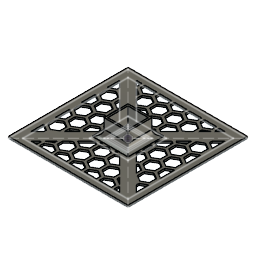
base (Autodesk Fusion 360 design; units mm, degrees)
Autodesk Fusion 360 part; units mm, degrees
(part 1 of 2)
sketch "Sketch4" plane through (0, 0, 0) normal (0, 0, 1) x (1, 0, 0)
  line L0 (100, -100) -> (-100, -100)
  line L1 (-100, -100) -> (-100, 100)
  line L2 (-100, 100) -> (100, 100)
  line L3 (100, 100) -> (100, -100)
  line L4 (100, -100) -> (-100, 100) construction
  line L5 (-100, -100) -> (100, 100) construction
  line L6 (20, -20) -> (-20, -20)
  line L7 (-20, -20) -> (-20, 20)
  line L8 (-20, 20) -> (20, 20)
  line L9 (20, 20) -> (20, -20)
  line L10 (20, -20) -> (-20, 20) construction
  line L11 (-20, -20) -> (20, 20) construction
  line L12 (-32, -32) -> (-32, 32)
  line L13 (-32, 32) -> (32, 32)
  line L14 (32, 32) -> (32, -32)
  line L15 (32, -32) -> (-32, -32)
  line L16 (88, -88) -> (-88, -88)
  line L17 (-88, -88) -> (-88, 88)
  line L18 (-88, 88) -> (88, 88)
  line L19 (88, 88) -> (88, -88)
  line L20 (17, 17) -> (17, -17)
  line L21 (17, -17) -> (-17, -17)
  line L22 (-17, -17) -> (-17, 17)
  line L23 (-17, 17) -> (17, 17)
  line L24 (14, -14) -> (-14, -14)
  line L25 (-14, -14) -> (-14, 14)
  line L26 (-14, 14) -> (14, 14)
  line L27 (14, 14) -> (14, -14)
  line L28 (-73.8579, 88) -> (-17.8579, 32)
  line L29 (-88, 73.8579) -> (-32, 17.8579)
  dimension "d22" = 200
  dimension "d23" = 200
  dimension "d24" = 40
  dimension "d25" = 40
  dimension "d26" = -12
  dimension "d27" = 12
  dimension "d44" = 3
  dimension "d49" = 6
  dimension "d50" = 20
  constraint horizontal L0
  constraint perpendicular L0 L1
  constraint parallel L0 L2
  constraint parallel L1 L3
  constraint coincident L4 origin
  constraint coincident L5 origin
  constraint horizontal L6
  constraint perpendicular L6 L7
  constraint parallel L6 L8
  constraint parallel L7 L9
  constraint coincident L10 origin
  constraint coincident L11 origin
  constraint coincident L18 L28.start
  constraint coincident L13 L28.end
  constraint coincident L17 L29.start
  constraint coincident L12 L29.end
  constraint parallel L4 L29
  constraint symmetric L4 L28 L29
  measures "d22" distance of L1.end L2.end
  measures "d23" distance of L0.end L1.end
  measures "d24" distance of L7.end L8.end
  measures "d25" distance of L6.end L7.end
  measures "d50" distance of L28 L29
extrude "Extrude4" add sketch "Sketch4" along normal blind 3 contours L0 L1 L2 L3 | L6 L7 L8 L9 | L12 L13 L14 L15 | L20 L21 L22 L23 | L24 L25 L26 L27 makes body 1 at (-96, -29.3333, 0) makes body 2 at (10.6667, -10.6667, 0)
sketch "Sketch6" plane through (0, 0, 0) normal (0, 0, 1) x (1, 0, 0)
  line L0 (10, 5.7735) -> (0, 11.547)
  line L1 (0, 11.547) -> (-10, 5.7735)
  line L2 (-10, 5.7735) -> (-10, -5.7735)
  line L3 (-10, -5.7735) -> (0, -11.547)
  line L4 (0, -11.547) -> (10, -5.7735)
  line L5 (10, -5.7735) -> (10, 5.7735)
  line L6 (0, 0) -> (10, 0) construction
  line L7 (0, 0) -> (5, -8.6603) construction
  line L8 (-237.5, 96.7062) -> (-227.5, 102.4797)
  line L9 (-227.5, 102.4797) -> (-227.5, 114.0267)
  line L10 (-227.5, 114.0267) -> (-237.5, 119.8002)
  line L11 (-237.5, 119.8002) -> (-247.5, 114.0267)
  line L12 (-247.5, 114.0267) -> (-247.5, 102.4797)
  line L13 (-247.5, 102.4797) -> (-237.5, 96.7062)
  line L14 (-212.5, 96.7062) -> (-202.5, 102.4797)
  line L15 (-202.5, 102.4797) -> (-202.5, 114.0267)
  line L16 (-202.5, 114.0267) -> (-212.5, 119.8002)
  line L17 (-212.5, 119.8002) -> (-222.5, 114.0267)
  line L18 (-222.5, 114.0267) -> (-222.5, 102.4797)
  line L19 (-222.5, 102.4797) -> (-212.5, 96.7062)
  line L20 (-187.5, 96.7062) -> (-177.5, 102.4797)
  line L21 (-177.5, 102.4797) -> (-177.5, 114.0267)
  line L22 (-177.5, 114.0267) -> (-187.5, 119.8002)
  line L23 (-187.5, 119.8002) -> (-197.5, 114.0267)
  line L24 (-197.5, 114.0267) -> (-197.5, 102.4797)
  line L25 (-197.5, 102.4797) -> (-187.5, 96.7062)
  line L26 (-162.5, 96.7062) -> (-152.5, 102.4797)
  line L27 (-152.5, 102.4797) -> (-152.5, 114.0267)
  line L28 (-152.5, 114.0267) -> (-162.5, 119.8002)
  line L29 (-162.5, 119.8002) -> (-172.5, 114.0267)
  line L30 (-172.5, 114.0267) -> (-172.5, 102.4797)
  line L31 (-172.5, 102.4797) -> (-162.5, 96.7062)
  line L32 (-137.5, 96.7062) -> (-127.5, 102.4797)
  line L33 (-127.5, 102.4797) -> (-127.5, 114.0267)
  line L34 (-127.5, 114.0267) -> (-137.5, 119.8002)
  line L35 (-137.5, 119.8002) -> (-147.5, 114.0267)
  line L36 (-147.5, 114.0267) -> (-147.5, 102.4797)
  line L37 (-147.5, 102.4797) -> (-137.5, 96.7062)
  line L38 (-112.5, 96.7062) -> (-102.5, 102.4797)
  line L39 (-102.5, 102.4797) -> (-102.5, 114.0267)
  line L40 (-102.5, 114.0267) -> (-112.5, 119.8002)
  line L41 (-112.5, 119.8002) -> (-122.5, 114.0267)
  line L42 (-122.5, 114.0267) -> (-122.5, 102.4797)
  line L43 (-122.5, 102.4797) -> (-112.5, 96.7062)
  line L44 (-87.5, 96.7062) -> (-77.5, 102.4797)
  line L45 (-77.5, 102.4797) -> (-77.5, 114.0267)
  line L46 (-77.5, 114.0267) -> (-87.5, 119.8002)
  line L47 (-87.5, 119.8002) -> (-97.5, 114.0267)
  line L48 (-97.5, 114.0267) -> (-97.5, 102.4797)
  line L49 (-97.5, 102.4797) -> (-87.5, 96.7062)
  line L50 (-62.5, 96.7062) -> (-52.5, 102.4797)
  line L51 (-52.5, 102.4797) -> (-52.5, 114.0267)
  line L52 (-52.5, 114.0267) -> (-62.5, 119.8002)
  line L53 (-62.5, 119.8002) -> (-72.5, 114.0267)
  line L54 (-72.5, 114.0267) -> (-72.5, 102.4797)
  line L55 (-72.5, 102.4797) -> (-62.5, 96.7062)
  line L56 (-37.5, 96.7062) -> (-27.5, 102.4797)
  line L57 (-27.5, 102.4797) -> (-27.5, 114.0267)
  line L58 (-27.5, 114.0267) -> (-37.5, 119.8002)
  line L59 (-37.5, 119.8002) -> (-47.5, 114.0267)
  line L60 (-47.5, 114.0267) -> (-47.5, 102.4797)
  line L61 (-47.5, 102.4797) -> (-37.5, 96.7062)
  line L62 (-12.5, 96.7062) -> (-2.5, 102.4797)
  line L63 (-2.5, 102.4797) -> (-2.5, 114.0267)
  line L64 (-2.5, 114.0267) -> (-12.5, 119.8002)
  line L65 (-12.5, 119.8002) -> (-22.5, 114.0267)
  line L66 (-22.5, 114.0267) -> (-22.5, 102.4797)
  line L67 (-22.5, 102.4797) -> (-12.5, 96.7062)
  line L68 (12.5, 96.7062) -> (22.5, 102.4797)
  line L69 (22.5, 102.4797) -> (22.5, 114.0267)
  line L70 (22.5, 114.0267) -> (12.5, 119.8002)
  line L71 (12.5, 119.8002) -> (2.5, 114.0267)
  line L72 (2.5, 114.0267) -> (2.5, 102.4797)
  line L73 (2.5, 102.4797) -> (12.5, 96.7062)
  line L74 (37.5, 96.7062) -> (47.5, 102.4797)
  line L75 (47.5, 102.4797) -> (47.5, 114.0267)
  line L76 (47.5, 114.0267) -> (37.5, 119.8002)
  line L77 (37.5, 119.8002) -> (27.5, 114.0267)
  line L78 (27.5, 114.0267) -> (27.5, 102.4797)
  line L79 (27.5, 102.4797) -> (37.5, 96.7062)
  line L80 (62.5, 96.7062) -> (72.5, 102.4797)
  line L81 (72.5, 102.4797) -> (72.5, 114.0267)
  line L82 (72.5, 114.0267) -> (62.5, 119.8002)
  line L83 (62.5, 119.8002) -> (52.5, 114.0267)
  line L84 (52.5, 114.0267) -> (52.5, 102.4797)
  line L85 (52.5, 102.4797) -> (62.5, 96.7062)
  line L86 (87.5, 96.7062) -> (97.5, 102.4797)
  line L87 (97.5, 102.4797) -> (97.5, 114.0267)
  line L88 (97.5, 114.0267) -> (87.5, 119.8002)
  line L89 (87.5, 119.8002) -> (77.5, 114.0267)
  line L90 (77.5, 114.0267) -> (77.5, 102.4797)
  line L91 (77.5, 102.4797) -> (87.5, 96.7062)
  line L92 (112.5, 96.7062) -> (122.5, 102.4797)
  line L93 (122.5, 102.4797) -> (122.5, 114.0267)
  line L94 (122.5, 114.0267) -> (112.5, 119.8002)
  line L95 (112.5, 119.8002) -> (102.5, 114.0267)
  line L96 (102.5, 114.0267) -> (102.5, 102.4797)
  line L97 (102.5, 102.4797) -> (112.5, 96.7062)
  line L98 (-225, 75.0555) -> (-215, 80.829)
  line L99 (-215, 80.829) -> (-215, 92.376)
  line L100 (-215, 92.376) -> (-225, 98.1495)
  line L101 (-225, 98.1495) -> (-235, 92.376)
  line L102 (-235, 92.376) -> (-235, 80.829)
  line L103 (-235, 80.829) -> (-225, 75.0555)
  line L104 (-200, 75.0555) -> (-190, 80.829)
  line L105 (-190, 80.829) -> (-190, 92.376)
  line L106 (-190, 92.376) -> (-200, 98.1495)
  line L107 (-200, 98.1495) -> (-210, 92.376)
  line L108 (-210, 92.376) -> (-210, 80.829)
  line L109 (-210, 80.829) -> (-200, 75.0555)
  line L110 (-175, 75.0555) -> (-165, 80.829)
  line L111 (-165, 80.829) -> (-165, 92.376)
  line L112 (-165, 92.376) -> (-175, 98.1495)
  line L113 (-175, 98.1495) -> (-185, 92.376)
  line L114 (-185, 92.376) -> (-185, 80.829)
  line L115 (-185, 80.829) -> (-175, 75.0555)
  line L116 (-150, 75.0555) -> (-140, 80.829)
  line L117 (-140, 80.829) -> (-140, 92.376)
  line L118 (-140, 92.376) -> (-150, 98.1495)
  line L119 (-150, 98.1495) -> (-160, 92.376)
  line L120 (-160, 92.376) -> (-160, 80.829)
  line L121 (-160, 80.829) -> (-150, 75.0555)
  line L122 (-125, 75.0555) -> (-115, 80.829)
  line L123 (-115, 80.829) -> (-115, 92.376)
  line L124 (-115, 92.376) -> (-125, 98.1495)
  line L125 (-125, 98.1495) -> (-135, 92.376)
  line L126 (-135, 92.376) -> (-135, 80.829)
  line L127 (-135, 80.829) -> (-125, 75.0555)
  line L128 (-100, 75.0555) -> (-90, 80.829)
  line L129 (-90, 80.829) -> (-90, 92.376)
  line L130 (-90, 92.376) -> (-100, 98.1495)
  line L131 (-100, 98.1495) -> (-110, 92.376)
  line L132 (-110, 92.376) -> (-110, 80.829)
  line L133 (-110, 80.829) -> (-100, 75.0555)
  line L134 (-75, 75.0555) -> (-65, 80.829)
  line L135 (-65, 80.829) -> (-65, 92.376)
  line L136 (-65, 92.376) -> (-75, 98.1495)
  line L137 (-75, 98.1495) -> (-85, 92.376)
  line L138 (-85, 92.376) -> (-85, 80.829)
  line L139 (-85, 80.829) -> (-75, 75.0555)
  line L140 (-50, 75.0555) -> (-40, 80.829)
  line L141 (-40, 80.829) -> (-40, 92.376)
  line L142 (-40, 92.376) -> (-50, 98.1495)
  line L143 (-50, 98.1495) -> (-60, 92.376)
  line L144 (-60, 92.376) -> (-60, 80.829)
  line L145 (-60, 80.829) -> (-50, 75.0555)
  line L146 (-25, 75.0555) -> (-15, 80.829)
  line L147 (-15, 80.829) -> (-15, 92.376)
  line L148 (-15, 92.376) -> (-25, 98.1495)
  line L149 (-25, 98.1495) -> (-35, 92.376)
  line L150 (-35, 92.376) -> (-35, 80.829)
  line L151 (-35, 80.829) -> (-25, 75.0555)
  line L152 (0, 75.0555) -> (10, 80.829)
  line L153 (10, 80.829) -> (10, 92.376)
  line L154 (10, 92.376) -> (0, 98.1495)
  line L155 (0, 98.1495) -> (-10, 92.376)
  line L156 (-10, 92.376) -> (-10, 80.829)
  line L157 (-10, 80.829) -> (0, 75.0555)
  line L158 (25, 75.0555) -> (35, 80.829)
  line L159 (35, 80.829) -> (35, 92.376)
  line L160 (35, 92.376) -> (25, 98.1495)
  line L161 (25, 98.1495) -> (15, 92.376)
  line L162 (15, 92.376) -> (15, 80.829)
  line L163 (15, 80.829) -> (25, 75.0555)
  line L164 (50, 75.0555) -> (60, 80.829)
  line L165 (60, 80.829) -> (60, 92.376)
  line L166 (60, 92.376) -> (50, 98.1495)
  line L167 (50, 98.1495) -> (40, 92.376)
  line L168 (40, 92.376) -> (40, 80.829)
  line L169 (40, 80.829) -> (50, 75.0555)
  line L170 (75, 75.0555) -> (85, 80.829)
  line L171 (85, 80.829) -> (85, 92.376)
  line L172 (85, 92.376) -> (75, 98.1495)
  line L173 (75, 98.1495) -> (65, 92.376)
  line L174 (65, 92.376) -> (65, 80.829)
  line L175 (65, 80.829) -> (75, 75.0555)
  line L176 (100, 75.0555) -> (110, 80.829)
  line L177 (110, 80.829) -> (110, 92.376)
  line L178 (110, 92.376) -> (100, 98.1495)
  line L179 (100, 98.1495) -> (90, 92.376)
  line L180 (90, 92.376) -> (90, 80.829)
  line L181 (90, 80.829) -> (100, 75.0555)
  line L182 (125, 75.0555) -> (135, 80.829)
  line L183 (135, 80.829) -> (135, 92.376)
  line L184 (135, 92.376) -> (125, 98.1495)
  line L185 (125, 98.1495) -> (115, 92.376)
  line L186 (115, 92.376) -> (115, 80.829)
  line L187 (115, 80.829) -> (125, 75.0555)
  line L188 (-212.5, 53.4049) -> (-202.5, 59.1784)
  line L189 (-202.5, 59.1784) -> (-202.5, 70.7254)
  line L190 (-202.5, 70.7254) -> (-212.5, 76.4989)
  line L191 (-212.5, 76.4989) -> (-222.5, 70.7254)
  line L192 (-222.5, 70.7254) -> (-222.5, 59.1784)
  line L193 (-222.5, 59.1784) -> (-212.5, 53.4049)
  line L194 (-187.5, 53.4049) -> (-177.5, 59.1784)
  line L195 (-177.5, 59.1784) -> (-177.5, 70.7254)
  line L196 (-177.5, 70.7254) -> (-187.5, 76.4989)
  line L197 (-187.5, 76.4989) -> (-197.5, 70.7254)
  line L198 (-197.5, 70.7254) -> (-197.5, 59.1784)
  line L199 (-197.5, 59.1784) -> (-187.5, 53.4049)
  line L200 (-162.5, 53.4049) -> (-152.5, 59.1784)
  line L201 (-152.5, 59.1784) -> (-152.5, 70.7254)
  line L202 (-152.5, 70.7254) -> (-162.5, 76.4989)
  line L203 (-162.5, 76.4989) -> (-172.5, 70.7254)
  line L204 (-172.5, 70.7254) -> (-172.5, 59.1784)
  line L205 (-172.5, 59.1784) -> (-162.5, 53.4049)
  line L206 (-137.5, 53.4049) -> (-127.5, 59.1784)
  line L207 (-127.5, 59.1784) -> (-127.5, 70.7254)
  line L208 (-127.5, 70.7254) -> (-137.5, 76.4989)
  line L209 (-137.5, 76.4989) -> (-147.5, 70.7254)
  line L210 (-147.5, 70.7254) -> (-147.5, 59.1784)
  line L211 (-147.5, 59.1784) -> (-137.5, 53.4049)
  line L212 (-112.5, 53.4049) -> (-102.5, 59.1784)
  line L213 (-102.5, 59.1784) -> (-102.5, 70.7254)
  line L214 (-102.5, 70.7254) -> (-112.5, 76.4989)
  line L215 (-112.5, 76.4989) -> (-122.5, 70.7254)
  line L216 (-122.5, 70.7254) -> (-122.5, 59.1784)
  line L217 (-122.5, 59.1784) -> (-112.5, 53.4049)
  line L218 (-87.5, 53.4049) -> (-77.5, 59.1784)
  line L219 (-77.5, 59.1784) -> (-77.5, 70.7254)
  line L220 (-77.5, 70.7254) -> (-87.5, 76.4989)
  line L221 (-87.5, 76.4989) -> (-97.5, 70.7254)
  line L222 (-97.5, 70.7254) -> (-97.5, 59.1784)
  line L223 (-97.5, 59.1784) -> (-87.5, 53.4049)
  line L224 (-62.5, 53.4049) -> (-52.5, 59.1784)
  line L225 (-52.5, 59.1784) -> (-52.5, 70.7254)
  line L226 (-52.5, 70.7254) -> (-62.5, 76.4989)
  line L227 (-62.5, 76.4989) -> (-72.5, 70.7254)
  line L228 (-72.5, 70.7254) -> (-72.5, 59.1784)
  line L229 (-72.5, 59.1784) -> (-62.5, 53.4049)
  line L230 (-37.5, 53.4049) -> (-27.5, 59.1784)
  line L231 (-27.5, 59.1784) -> (-27.5, 70.7254)
  line L232 (-27.5, 70.7254) -> (-37.5, 76.4989)
  line L233 (-37.5, 76.4989) -> (-47.5, 70.7254)
  line L234 (-47.5, 70.7254) -> (-47.5, 59.1784)
  line L235 (-47.5, 59.1784) -> (-37.5, 53.4049)
  line L236 (-12.5, 53.4049) -> (-2.5, 59.1784)
  line L237 (-2.5, 59.1784) -> (-2.5, 70.7254)
  line L238 (-2.5, 70.7254) -> (-12.5, 76.4989)
  line L239 (-12.5, 76.4989) -> (-22.5, 70.7254)
  line L240 (-22.5, 70.7254) -> (-22.5, 59.1784)
  line L241 (-22.5, 59.1784) -> (-12.5, 53.4049)
  line L242 (12.5, 53.4049) -> (22.5, 59.1784)
  line L243 (22.5, 59.1784) -> (22.5, 70.7254)
  line L244 (22.5, 70.7254) -> (12.5, 76.4989)
  line L245 (12.5, 76.4989) -> (2.5, 70.7254)
  line L246 (2.5, 70.7254) -> (2.5, 59.1784)
  line L247 (2.5, 59.1784) -> (12.5, 53.4049)
  line L248 (37.5, 53.4049) -> (47.5, 59.1784)
  line L249 (47.5, 59.1784) -> (47.5, 70.7254)
  line L250 (47.5, 70.7254) -> (37.5, 76.4989)
  line L251 (37.5, 76.4989) -> (27.5, 70.7254)
  line L252 (27.5, 70.7254) -> (27.5, 59.1784)
  line L253 (27.5, 59.1784) -> (37.5, 53.4049)
  line L254 (62.5, 53.4049) -> (72.5, 59.1784)
  line L255 (72.5, 59.1784) -> (72.5, 70.7254)
  line L256 (72.5, 70.7254) -> (62.5, 76.4989)
  line L257 (62.5, 76.4989) -> (52.5, 70.7254)
  line L258 (52.5, 70.7254) -> (52.5, 59.1784)
  line L259 (52.5, 59.1784) -> (62.5, 53.4049)
  line L260 (87.5, 53.4049) -> (97.5, 59.1784)
  line L261 (97.5, 59.1784) -> (97.5, 70.7254)
  line L262 (97.5, 70.7254) -> (87.5, 76.4989)
  line L263 (87.5, 76.4989) -> (77.5, 70.7254)
  line L264 (77.5, 70.7254) -> (77.5, 59.1784)
  line L265 (77.5, 59.1784) -> (87.5, 53.4049)
  line L266 (112.5, 53.4049) -> (122.5, 59.1784)
  line L267 (122.5, 59.1784) -> (122.5, 70.7254)
  line L268 (122.5, 70.7254) -> (112.5, 76.4989)
  line L269 (112.5, 76.4989) -> (102.5, 70.7254)
  line L270 (102.5, 70.7254) -> (102.5, 59.1784)
  line L271 (102.5, 59.1784) -> (112.5, 53.4049)
  line L272 (137.5, 53.4049) -> (147.5, 59.1784)
  line L273 (147.5, 59.1784) -> (147.5, 70.7254)
  line L274 (147.5, 70.7254) -> (137.5, 76.4989)
  line L275 (137.5, 76.4989) -> (127.5, 70.7254)
  line L276 (127.5, 70.7254) -> (127.5, 59.1784)
  line L277 (127.5, 59.1784) -> (137.5, 53.4049)
  line L278 (-200, 31.7543) -> (-190, 37.5278)
  line L279 (-190, 37.5278) -> (-190, 49.0748)
  line L280 (-190, 49.0748) -> (-200, 54.8483)
  line L281 (-200, 54.8483) -> (-210, 49.0748)
  line L282 (-210, 49.0748) -> (-210, 37.5278)
  line L283 (-210, 37.5278) -> (-200, 31.7543)
  line L284 (-175, 31.7543) -> (-165, 37.5278)
  line L285 (-165, 37.5278) -> (-165, 49.0748)
  line L286 (-165, 49.0748) -> (-175, 54.8483)
  line L287 (-175, 54.8483) -> (-185, 49.0748)
  line L288 (-185, 49.0748) -> (-185, 37.5278)
  line L289 (-185, 37.5278) -> (-175, 31.7543)
  line L290 (-150, 31.7543) -> (-140, 37.5278)
  line L291 (-140, 37.5278) -> (-140, 49.0748)
  line L292 (-140, 49.0748) -> (-150, 54.8483)
  line L293 (-150, 54.8483) -> (-160, 49.0748)
  line L294 (-160, 49.0748) -> (-160, 37.5278)
  line L295 (-160, 37.5278) -> (-150, 31.7543)
  line L296 (-125, 31.7543) -> (-115, 37.5278)
  line L297 (-115, 37.5278) -> (-115, 49.0748)
  line L298 (-115, 49.0748) -> (-125, 54.8483)
  line L299 (-125, 54.8483) -> (-135, 49.0748)
  line L300 (-135, 49.0748) -> (-135, 37.5278)
  line L301 (-135, 37.5278) -> (-125, 31.7543)
  line L302 (-100, 31.7543) -> (-90, 37.5278)
  line L303 (-90, 37.5278) -> (-90, 49.0748)
  line L304 (-90, 49.0748) -> (-100, 54.8483)
  line L305 (-100, 54.8483) -> (-110, 49.0748)
  line L306 (-110, 49.0748) -> (-110, 37.5278)
  line L307 (-110, 37.5278) -> (-100, 31.7543)
  line L308 (-75, 31.7543) -> (-65, 37.5278)
  line L309 (-65, 37.5278) -> (-65, 49.0748)
  line L310 (-65, 49.0748) -> (-75, 54.8483)
  line L311 (-75, 54.8483) -> (-85, 49.0748)
  line L312 (-85, 49.0748) -> (-85, 37.5278)
  line L313 (-85, 37.5278) -> (-75, 31.7543)
  line L314 (-50, 31.7543) -> (-40, 37.5278)
  line L315 (-40, 37.5278) -> (-40, 49.0748)
  line L316 (-40, 49.0748) -> (-50, 54.8483)
  line L317 (-50, 54.8483) -> (-60, 49.0748)
  line L318 (-60, 49.0748) -> (-60, 37.5278)
  line L319 (-60, 37.5278) -> (-50, 31.7543)
  line L320 (-25, 31.7543) -> (-15, 37.5278)
  line L321 (-15, 37.5278) -> (-15, 49.0748)
  line L322 (-15, 49.0748) -> (-25, 54.8483)
  line L323 (-25, 54.8483) -> (-35, 49.0748)
  line L324 (-35, 49.0748) -> (-35, 37.5278)
  line L325 (-35, 37.5278) -> (-25, 31.7543)
  line L326 (0, 31.7543) -> (10, 37.5278)
  line L327 (10, 37.5278) -> (10, 49.0748)
  line L328 (10, 49.0748) -> (0, 54.8483)
  line L329 (0, 54.8483) -> (-10, 49.0748)
  line L330 (-10, 49.0748) -> (-10, 37.5278)
  line L331 (-10, 37.5278) -> (0, 31.7543)
  line L332 (25, 31.7543) -> (35, 37.5278)
  line L333 (35, 37.5278) -> (35, 49.0748)
  line L334 (35, 49.0748) -> (25, 54.8483)
  line L335 (25, 54.8483) -> (15, 49.0748)
  line L336 (15, 49.0748) -> (15, 37.5278)
  line L337 (15, 37.5278) -> (25, 31.7543)
  line L338 (50, 31.7543) -> (60, 37.5278)
  line L339 (60, 37.5278) -> (60, 49.0748)
  line L340 (60, 49.0748) -> (50, 54.8483)
  line L341 (50, 54.8483) -> (40, 49.0748)
  line L342 (40, 49.0748) -> (40, 37.5278)
  line L343 (40, 37.5278) -> (50, 31.7543)
  line L344 (75, 31.7543) -> (85, 37.5278)
  line L345 (85, 37.5278) -> (85, 49.0748)
  line L346 (85, 49.0748) -> (75, 54.8483)
  line L347 (75, 54.8483) -> (65, 49.0748)
  line L348 (65, 49.0748) -> (65, 37.5278)
  line L349 (65, 37.5278) -> (75, 31.7543)
  line L350 (100, 31.7543) -> (110, 37.5278)
  line L351 (110, 37.5278) -> (110, 49.0748)
  line L352 (110, 49.0748) -> (100, 54.8483)
  line L353 (100, 54.8483) -> (90, 49.0748)
  line L354 (90, 49.0748) -> (90, 37.5278)
  line L355 (90, 37.5278) -> (100, 31.7543)
  line L356 (125, 31.7543) -> (135, 37.5278)
  line L357 (135, 37.5278) -> (135, 49.0748)
  line L358 (135, 49.0748) -> (125, 54.8483)
  line L359 (125, 54.8483) -> (115, 49.0748)
  line L360 (115, 49.0748) -> (115, 37.5278)
  line L361 (115, 37.5278) -> (125, 31.7543)
  line L362 (150, 31.7543) -> (160, 37.5278)
  line L363 (160, 37.5278) -> (160, 49.0748)
  line L364 (160, 49.0748) -> (150, 54.8483)
  line L365 (150, 54.8483) -> (140, 49.0748)
  line L366 (140, 49.0748) -> (140, 37.5278)
  line L367 (140, 37.5278) -> (150, 31.7543)
  line L368 (-187.5, 10.1036) -> (-177.5, 15.8771)
  line L369 (-177.5, 15.8771) -> (-177.5, 27.4241)
  line L370 (-177.5, 27.4241) -> (-187.5, 33.1976)
  line L371 (-187.5, 33.1976) -> (-197.5, 27.4241)
  line L372 (-197.5, 27.4241) -> (-197.5, 15.8771)
  line L373 (-197.5, 15.8771) -> (-187.5, 10.1036)
  line L374 (-162.5, 10.1036) -> (-152.5, 15.8771)
  line L375 (-152.5, 15.8771) -> (-152.5, 27.4241)
  line L376 (-152.5, 27.4241) -> (-162.5, 33.1976)
  line L377 (-162.5, 33.1976) -> (-172.5, 27.4241)
  line L378 (-172.5, 27.4241) -> (-172.5, 15.8771)
  line L379 (-172.5, 15.8771) -> (-162.5, 10.1036)
  line L380 (-137.5, 10.1036) -> (-127.5, 15.8771)
  line L381 (-127.5, 15.8771) -> (-127.5, 27.4241)
  line L382 (-127.5, 27.4241) -> (-137.5, 33.1976)
  line L383 (-137.5, 33.1976) -> (-147.5, 27.4241)
  line L384 (-147.5, 27.4241) -> (-147.5, 15.8771)
  line L385 (-147.5, 15.8771) -> (-137.5, 10.1036)
  line L386 (-112.5, 10.1036) -> (-102.5, 15.8771)
  line L387 (-102.5, 15.8771) -> (-102.5, 27.4241)
  line L388 (-102.5, 27.4241) -> (-112.5, 33.1976)
  line L389 (-112.5, 33.1976) -> (-122.5, 27.4241)
  line L390 (-122.5, 27.4241) -> (-122.5, 15.8771)
  line L391 (-122.5, 15.8771) -> (-112.5, 10.1036)
  line L392 (-87.5, 10.1036) -> (-77.5, 15.8771)
  line L393 (-77.5, 15.8771) -> (-77.5, 27.4241)
  line L394 (-77.5, 27.4241) -> (-87.5, 33.1976)
  line L395 (-87.5, 33.1976) -> (-97.5, 27.4241)
  line L396 (-97.5, 27.4241) -> (-97.5, 15.8771)
  line L397 (-97.5, 15.8771) -> (-87.5, 10.1036)
  line L398 (-62.5, 10.1036) -> (-52.5, 15.8771)
  line L399 (-52.5, 15.8771) -> (-52.5, 27.4241)
  line L400 (-52.5, 27.4241) -> (-62.5, 33.1976)
  line L401 (-62.5, 33.1976) -> (-72.5, 27.4241)
  line L402 (-72.5, 27.4241) -> (-72.5, 15.8771)
  line L403 (-72.5, 15.8771) -> (-62.5, 10.1036)
  line L404 (-37.5, 10.1036) -> (-27.5, 15.8771)
  line L405 (-27.5, 15.8771) -> (-27.5, 27.4241)
  line L406 (-27.5, 27.4241) -> (-37.5, 33.1976)
  line L407 (-37.5, 33.1976) -> (-47.5, 27.4241)
  line L408 (-47.5, 27.4241) -> (-47.5, 15.8771)
  line L409 (-47.5, 15.8771) -> (-37.5, 10.1036)
  line L410 (-12.5, 10.1036) -> (-2.5, 15.8771)
  line L411 (-2.5, 15.8771) -> (-2.5, 27.4241)
  line L412 (-2.5, 27.4241) -> (-12.5, 33.1976)
  line L413 (-12.5, 33.1976) -> (-22.5, 27.4241)
  line L414 (-22.5, 27.4241) -> (-22.5, 15.8771)
  line L415 (-22.5, 15.8771) -> (-12.5, 10.1036)
  line L416 (12.5, 10.1036) -> (22.5, 15.8771)
  line L417 (22.5, 15.8771) -> (22.5, 27.4241)
  line L418 (22.5, 27.4241) -> (12.5, 33.1976)
  line L419 (12.5, 33.1976) -> (2.5, 27.4241)
  line L420 (2.5, 27.4241) -> (2.5, 15.8771)
  line L421 (2.5, 15.8771) -> (12.5, 10.1036)
  line L422 (37.5, 10.1036) -> (47.5, 15.8771)
  line L423 (47.5, 15.8771) -> (47.5, 27.4241)
  line L424 (47.5, 27.4241) -> (37.5, 33.1976)
  line L425 (37.5, 33.1976) -> (27.5, 27.4241)
  line L426 (27.5, 27.4241) -> (27.5, 15.8771)
  line L427 (27.5, 15.8771) -> (37.5, 10.1036)
  line L428 (62.5, 10.1036) -> (72.5, 15.8771)
  line L429 (72.5, 15.8771) -> (72.5, 27.4241)
  line L430 (72.5, 27.4241) -> (62.5, 33.1976)
  line L431 (62.5, 33.1976) -> (52.5, 27.4241)
  line L432 (52.5, 27.4241) -> (52.5, 15.8771)
  line L433 (52.5, 15.8771) -> (62.5, 10.1036)
  line L434 (87.5, 10.1036) -> (97.5, 15.8771)
  line L435 (97.5, 15.8771) -> (97.5, 27.4241)
  line L436 (97.5, 27.4241) -> (87.5, 33.1976)
  line L437 (87.5, 33.1976) -> (77.5, 27.4241)
  line L438 (77.5, 27.4241) -> (77.5, 15.8771)
  line L439 (77.5, 15.8771) -> (87.5, 10.1036)
  line L440 (112.5, 10.1036) -> (122.5, 15.8771)
  line L441 (122.5, 15.8771) -> (122.5, 27.4241)
  line L442 (122.5, 27.4241) -> (112.5, 33.1976)
  line L443 (112.5, 33.1976) -> (102.5, 27.4241)
  line L444 (102.5, 27.4241) -> (102.5, 15.8771)
  line L445 (102.5, 15.8771) -> (112.5, 10.1036)
  line L446 (137.5, 10.1036) -> (147.5, 15.8771)
  line L447 (147.5, 15.8771) -> (147.5, 27.4241)
  line L448 (147.5, 27.4241) -> (137.5, 33.1976)
  line L449 (137.5, 33.1976) -> (127.5, 27.4241)
  line L450 (127.5, 27.4241) -> (127.5, 15.8771)
  line L451 (127.5, 15.8771) -> (137.5, 10.1036)
  line L452 (162.5, 10.1036) -> (172.5, 15.8771)
  line L453 (172.5, 15.8771) -> (172.5, 27.4241)
  line L454 (172.5, 27.4241) -> (162.5, 33.1976)
  line L455 (162.5, 33.1976) -> (152.5, 27.4241)
  line L456 (152.5, 27.4241) -> (152.5, 15.8771)
  line L457 (152.5, 15.8771) -> (162.5, 10.1036)
  line L458 (-175, -11.547) -> (-165, -5.7735)
  line L459 (-165, -5.7735) -> (-165, 5.7735)
  line L460 (-165, 5.7735) -> (-175, 11.547)
  line L461 (-175, 11.547) -> (-185, 5.7735)
  line L462 (-185, 5.7735) -> (-185, -5.7735)
  line L463 (-185, -5.7735) -> (-175, -11.547)
  line L464 (-150, -11.547) -> (-140, -5.7735)
  line L465 (-140, -5.7735) -> (-140, 5.7735)
  line L466 (-140, 5.7735) -> (-150, 11.547)
  line L467 (-150, 11.547) -> (-160, 5.7735)
  line L468 (-160, 5.7735) -> (-160, -5.7735)
  line L469 (-160, -5.7735) -> (-150, -11.547)
  line L470 (-125, -11.547) -> (-115, -5.7735)
  line L471 (-115, -5.7735) -> (-115, 5.7735)
  line L472 (-115, 5.7735) -> (-125, 11.547)
  line L473 (-125, 11.547) -> (-135, 5.7735)
  line L474 (-135, 5.7735) -> (-135, -5.7735)
  line L475 (-135, -5.7735) -> (-125, -11.547)
  line L476 (-100, -11.547) -> (-90, -5.7735)
  line L477 (-90, -5.7735) -> (-90, 5.7735)
  line L478 (-90, 5.7735) -> (-100, 11.547)
  line L479 (-100, 11.547) -> (-110, 5.7735)
  line L480 (-110, 5.7735) -> (-110, -5.7735)
  line L481 (-110, -5.7735) -> (-100, -11.547)
  line L482 (-75, -11.547) -> (-65, -5.7735)
  line L483 (-65, -5.7735) -> (-65, 5.7735)
  line L484 (-65, 5.7735) -> (-75, 11.547)
  line L485 (-75, 11.547) -> (-85, 5.7735)
  line L486 (-85, 5.7735) -> (-85, -5.7735)
  line L487 (-85, -5.7735) -> (-75, -11.547)
  line L488 (-50, -11.547) -> (-40, -5.7735)
  line L489 (-40, -5.7735) -> (-40, 5.7735)
  line L490 (-40, 5.7735) -> (-50, 11.547)
  line L491 (-50, 11.547) -> (-60, 5.7735)
  line L492 (-60, 5.7735) -> (-60, -5.7735)
  line L493 (-60, -5.7735) -> (-50, -11.547)
  line L494 (-25, -11.547) -> (-15, -5.7735)
  line L495 (-15, -5.7735) -> (-15, 5.7735)
  line L496 (-15, 5.7735) -> (-25, 11.547)
  line L497 (-25, 11.547) -> (-35, 5.7735)
  line L498 (-35, 5.7735) -> (-35, -5.7735)
  line L499 (-35, -5.7735) -> (-25, -11.547)
  line L500 (25, -11.547) -> (35, -5.7735)
  line L501 (35, -5.7735) -> (35, 5.7735)
  line L502 (35, 5.7735) -> (25, 11.547)
  line L503 (25, 11.547) -> (15, 5.7735)
  line L504 (15, 5.7735) -> (15, -5.7735)
  line L505 (15, -5.7735) -> (25, -11.547)
  line L506 (50, -11.547) -> (60, -5.7735)
  line L507 (60, -5.7735) -> (60, 5.7735)
  line L508 (60, 5.7735) -> (50, 11.547)
  line L509 (50, 11.547) -> (40, 5.7735)
  line L510 (40, 5.7735) -> (40, -5.7735)
  line L511 (40, -5.7735) -> (50, -11.547)
  line L512 (75, -11.547) -> (85, -5.7735)
  line L513 (85, -5.7735) -> (85, 5.7735)
  line L514 (85, 5.7735) -> (75, 11.547)
  line L515 (75, 11.547) -> (65, 5.7735)
  line L516 (65, 5.7735) -> (65, -5.7735)
  line L517 (65, -5.7735) -> (75, -11.547)
  line L518 (100, -11.547) -> (110, -5.7735)
  line L519 (110, -5.7735) -> (110, 5.7735)
  line L520 (110, 5.7735) -> (100, 11.547)
  line L521 (100, 11.547) -> (90, 5.7735)
  line L522 (90, 5.7735) -> (90, -5.7735)
  line L523 (90, -5.7735) -> (100, -11.547)
  line L524 (125, -11.547) -> (135, -5.7735)
  line L525 (135, -5.7735) -> (135, 5.7735)
  line L526 (135, 5.7735) -> (125, 11.547)
  line L527 (125, 11.547) -> (115, 5.7735)
  line L528 (115, 5.7735) -> (115, -5.7735)
  line L529 (115, -5.7735) -> (125, -11.547)
  line L530 (150, -11.547) -> (160, -5.7735)
  line L531 (160, -5.7735) -> (160, 5.7735)
  line L532 (160, 5.7735) -> (150, 11.547)
  line L533 (150, 11.547) -> (140, 5.7735)
  line L534 (140, 5.7735) -> (140, -5.7735)
  line L535 (140, -5.7735) -> (150, -11.547)
  line L536 (175, -11.547) -> (185, -5.7735)
  line L537 (185, -5.7735) -> (185, 5.7735)
  line L538 (185, 5.7735) -> (175, 11.547)
  line L539 (175, 11.547) -> (165, 5.7735)
  line L540 (165, 5.7735) -> (165, -5.7735)
  line L541 (165, -5.7735) -> (175, -11.547)
  line L542 (-162.5, -33.1976) -> (-152.5, -27.4241)
  line L543 (-152.5, -27.4241) -> (-152.5, -15.8771)
  line L544 (-152.5, -15.8771) -> (-162.5, -10.1036)
  line L545 (-162.5, -10.1036) -> (-172.5, -15.8771)
  line L546 (-172.5, -15.8771) -> (-172.5, -27.4241)
  line L547 (-172.5, -27.4241) -> (-162.5, -33.1976)
  line L548 (-137.5, -33.1976) -> (-127.5, -27.4241)
  line L549 (-127.5, -27.4241) -> (-127.5, -15.8771)
  line L550 (-127.5, -15.8771) -> (-137.5, -10.1036)
  line L551 (-137.5, -10.1036) -> (-147.5, -15.8771)
  line L552 (-147.5, -15.8771) -> (-147.5, -27.4241)
  line L553 (-147.5, -27.4241) -> (-137.5, -33.1976)
  line L554 (-112.5, -33.1976) -> (-102.5, -27.4241)
  line L555 (-102.5, -27.4241) -> (-102.5, -15.8771)
  line L556 (-102.5, -15.8771) -> (-112.5, -10.1036)
  line L557 (-112.5, -10.1036) -> (-122.5, -15.8771)
  line L558 (-122.5, -15.8771) -> (-122.5, -27.4241)
  line L559 (-122.5, -27.4241) -> (-112.5, -33.1976)
  line L560 (-87.5, -33.1976) -> (-77.5, -27.4241)
  line L561 (-77.5, -27.4241) -> (-77.5, -15.8771)
  line L562 (-77.5, -15.8771) -> (-87.5, -10.1036)
  line L563 (-87.5, -10.1036) -> (-97.5, -15.8771)
  line L564 (-97.5, -15.8771) -> (-97.5, -27.4241)
  line L565 (-97.5, -27.4241) -> (-87.5, -33.1976)
  line L566 (-62.5, -33.1976) -> (-52.5, -27.4241)
  line L567 (-52.5, -27.4241) -> (-52.5, -15.8771)
  line L568 (-52.5, -15.8771) -> (-62.5, -10.1036)
  line L569 (-62.5, -10.1036) -> (-72.5, -15.8771)
  line L570 (-72.5, -15.8771) -> (-72.5, -27.4241)
  line L571 (-72.5, -27.4241) -> (-62.5, -33.1976)
  line L572 (-37.5, -33.1976) -> (-27.5, -27.4241)
  line L573 (-27.5, -27.4241) -> (-27.5, -15.8771)
  line L574 (-27.5, -15.8771) -> (-37.5, -10.1036)
  line L575 (-37.5, -10.1036) -> (-47.5, -15.8771)
  line L576 (-47.5, -15.8771) -> (-47.5, -27.4241)
  line L577 (-47.5, -27.4241) -> (-37.5, -33.1976)
  line L578 (-12.5, -33.1976) -> (-2.5, -27.4241)
  line L579 (-2.5, -27.4241) -> (-2.5, -15.8771)
  line L580 (-2.5, -15.8771) -> (-12.5, -10.1036)
  line L581 (-12.5, -10.1036) -> (-22.5, -15.8771)
  line L582 (-22.5, -15.8771) -> (-22.5, -27.4241)
  line L583 (-22.5, -27.4241) -> (-12.5, -33.1976)
  line L584 (12.5, -33.1976) -> (22.5, -27.4241)
  line L585 (22.5, -27.4241) -> (22.5, -15.8771)
  line L586 (22.5, -15.8771) -> (12.5, -10.1036)
  line L587 (12.5, -10.1036) -> (2.5, -15.8771)
  line L588 (2.5, -15.8771) -> (2.5, -27.4241)
  line L589 (2.5, -27.4241) -> (12.5, -33.1976)
  line L590 (37.5, -33.1976) -> (47.5, -27.4241)
  line L591 (47.5, -27.4241) -> (47.5, -15.8771)
  line L592 (47.5, -15.8771) -> (37.5, -10.1036)
  line L593 (37.5, -10.1036) -> (27.5, -15.8771)
  line L594 (27.5, -15.8771) -> (27.5, -27.4241)
  line L595 (27.5, -27.4241) -> (37.5, -33.1976)
  line L596 (62.5, -33.1976) -> (72.5, -27.4241)
  line L597 (72.5, -27.4241) -> (72.5, -15.8771)
  line L598 (72.5, -15.8771) -> (62.5, -10.1036)
  line L599 (62.5, -10.1036) -> (52.5, -15.8771)
  line L600 (52.5, -15.8771) -> (52.5, -27.4241)
  line L601 (52.5, -27.4241) -> (62.5, -33.1976)
  line L602 (87.5, -33.1976) -> (97.5, -27.4241)
  line L603 (97.5, -27.4241) -> (97.5, -15.8771)
  line L604 (97.5, -15.8771) -> (87.5, -10.1036)
  line L605 (87.5, -10.1036) -> (77.5, -15.8771)
  line L606 (77.5, -15.8771) -> (77.5, -27.4241)
  line L607 (77.5, -27.4241) -> (87.5, -33.1976)
  line L608 (112.5, -33.1976) -> (122.5, -27.4241)
  line L609 (122.5, -27.4241) -> (122.5, -15.8771)
  line L610 (122.5, -15.8771) -> (112.5, -10.1036)
  line L611 (112.5, -10.1036) -> (102.5, -15.8771)
  line L612 (102.5, -15.8771) -> (102.5, -27.4241)
  line L613 (102.5, -27.4241) -> (112.5, -33.1976)
  line L614 (137.5, -33.1976) -> (147.5, -27.4241)
  line L615 (147.5, -27.4241) -> (147.5, -15.8771)
  line L616 (147.5, -15.8771) -> (137.5, -10.1036)
  line L617 (137.5, -10.1036) -> (127.5, -15.8771)
  line L618 (127.5, -15.8771) -> (127.5, -27.4241)
  line L619 (127.5, -27.4241) -> (137.5, -33.1976)
  line L620 (162.5, -33.1976) -> (172.5, -27.4241)
  line L621 (172.5, -27.4241) -> (172.5, -15.8771)
  line L622 (172.5, -15.8771) -> (162.5, -10.1036)
  line L623 (162.5, -10.1036) -> (152.5, -15.8771)
  line L624 (152.5, -15.8771) -> (152.5, -27.4241)
  line L625 (152.5, -27.4241) -> (162.5, -33.1976)
  line L626 (187.5, -33.1976) -> (197.5, -27.4241)
  line L627 (197.5, -27.4241) -> (197.5, -15.8771)
  line L628 (197.5, -15.8771) -> (187.5, -10.1036)
  line L629 (187.5, -10.1036) -> (177.5, -15.8771)
  line L630 (177.5, -15.8771) -> (177.5, -27.4241)
  line L631 (177.5, -27.4241) -> (187.5, -33.1976)
  line L632 (-150, -54.8483) -> (-140, -49.0748)
  line L633 (-140, -49.0748) -> (-140, -37.5278)
  line L634 (-140, -37.5278) -> (-150, -31.7543)
  line L635 (-150, -31.7543) -> (-160, -37.5278)
  line L636 (-160, -37.5278) -> (-160, -49.0748)
  line L637 (-160, -49.0748) -> (-150, -54.8483)
  line L638 (-125, -54.8483) -> (-115, -49.0748)
  line L639 (-115, -49.0748) -> (-115, -37.5278)
  line L640 (-115, -37.5278) -> (-125, -31.7543)
  line L641 (-125, -31.7543) -> (-135, -37.5278)
  line L642 (-135, -37.5278) -> (-135, -49.0748)
  line L643 (-135, -49.0748) -> (-125, -54.8483)
  line L644 (-100, -54.8483) -> (-90, -49.0748)
  line L645 (-90, -49.0748) -> (-90, -37.5278)
  line L646 (-90, -37.5278) -> (-100, -31.7543)
  line L647 (-100, -31.7543) -> (-110, -37.5278)
  line L648 (-110, -37.5278) -> (-110, -49.0748)
  line L649 (-110, -49.0748) -> (-100, -54.8483)
  line L650 (-75, -54.8483) -> (-65, -49.0748)
  line L651 (-65, -49.0748) -> (-65, -37.5278)
  line L652 (-65, -37.5278) -> (-75, -31.7543)
  line L653 (-75, -31.7543) -> (-85, -37.5278)
  line L654 (-85, -37.5278) -> (-85, -49.0748)
  line L655 (-85, -49.0748) -> (-75, -54.8483)
  line L656 (-50, -54.8483) -> (-40, -49.0748)
  line L657 (-40, -49.0748) -> (-40, -37.5278)
  line L658 (-40, -37.5278) -> (-50, -31.7543)
  line L659 (-50, -31.7543) -> (-60, -37.5278)
  line L660 (-60, -37.5278) -> (-60, -49.0748)
  line L661 (-60, -49.0748) -> (-50, -54.8483)
  line L662 (-25, -54.8483) -> (-15, -49.0748)
  line L663 (-15, -49.0748) -> (-15, -37.5278)
  line L664 (-15, -37.5278) -> (-25, -31.7543)
  line L665 (-25, -31.7543) -> (-35, -37.5278)
  line L666 (-35, -37.5278) -> (-35, -49.0748)
  line L667 (-35, -49.0748) -> (-25, -54.8483)
  line L668 (0, -54.8483) -> (10, -49.0748)
  line L669 (10, -49.0748) -> (10, -37.5278)
  line L670 (10, -37.5278) -> (0, -31.7543)
  line L671 (0, -31.7543) -> (-10, -37.5278)
  line L672 (-10, -37.5278) -> (-10, -49.0748)
  line L673 (-10, -49.0748) -> (0, -54.8483)
  line L674 (25, -54.8483) -> (35, -49.0748)
  line L675 (35, -49.0748) -> (35, -37.5278)
  line L676 (35, -37.5278) -> (25, -31.7543)
  line L677 (25, -31.7543) -> (15, -37.5278)
  line L678 (15, -37.5278) -> (15, -49.0748)
  line L679 (15, -49.0748) -> (25, -54.8483)
  line L680 (50, -54.8483) -> (60, -49.0748)
  line L681 (60, -49.0748) -> (60, -37.5278)
  line L682 (60, -37.5278) -> (50, -31.7543)
  line L683 (50, -31.7543) -> (40, -37.5278)
  line L684 (40, -37.5278) -> (40, -49.0748)
  line L685 (40, -49.0748) -> (50, -54.8483)
  line L686 (75, -54.8483) -> (85, -49.0748)
  line L687 (85, -49.0748) -> (85, -37.5278)
  line L688 (85, -37.5278) -> (75, -31.7543)
  line L689 (75, -31.7543) -> (65, -37.5278)
  line L690 (65, -37.5278) -> (65, -49.0748)
  line L691 (65, -49.0748) -> (75, -54.8483)
  line L692 (100, -54.8483) -> (110, -49.0748)
  line L693 (110, -49.0748) -> (110, -37.5278)
  line L694 (110, -37.5278) -> (100, -31.7543)
  line L695 (100, -31.7543) -> (90, -37.5278)
  line L696 (90, -37.5278) -> (90, -49.0748)
  line L697 (90, -49.0748) -> (100, -54.8483)
  line L698 (125, -54.8483) -> (135, -49.0748)
  line L699 (135, -49.0748) -> (135, -37.5278)
  line L700 (135, -37.5278) -> (125, -31.7543)
  line L701 (125, -31.7543) -> (115, -37.5278)
  line L702 (115, -37.5278) -> (115, -49.0748)
  line L703 (115, -49.0748) -> (125, -54.8483)
  line L704 (150, -54.8483) -> (160, -49.0748)
  line L705 (160, -49.0748) -> (160, -37.5278)
  line L706 (160, -37.5278) -> (150, -31.7543)
  line L707 (150, -31.7543) -> (140, -37.5278)
  line L708 (140, -37.5278) -> (140, -49.0748)
  line L709 (140, -49.0748) -> (150, -54.8483)
  line L710 (175, -54.8483) -> (185, -49.0748)
  line L711 (185, -49.0748) -> (185, -37.5278)
  line L712 (185, -37.5278) -> (175, -31.7543)
  line L713 (175, -31.7543) -> (165, -37.5278)
  line L714 (165, -37.5278) -> (165, -49.0748)
  line L715 (165, -49.0748) -> (175, -54.8483)
  line L716 (200, -54.8483) -> (210, -49.0748)
  line L717 (210, -49.0748) -> (210, -37.5278)
  line L718 (210, -37.5278) -> (200, -31.7543)
  line L719 (200, -31.7543) -> (190, -37.5278)
  line L720 (190, -37.5278) -> (190, -49.0748)
  line L721 (190, -49.0748) -> (200, -54.8483)
  line L722 (-137.5, -76.4989) -> (-127.5, -70.7254)
  line L723 (-127.5, -70.7254) -> (-127.5, -59.1784)
  line L724 (-127.5, -59.1784) -> (-137.5, -53.4049)
  line L725 (-137.5, -53.4049) -> (-147.5, -59.1784)
  line L726 (-147.5, -59.1784) -> (-147.5, -70.7254)
  line L727 (-147.5, -70.7254) -> (-137.5, -76.4989)
  line L728 (-112.5, -76.4989) -> (-102.5, -70.7254)
  line L729 (-102.5, -70.7254) -> (-102.5, -59.1784)
  line L730 (-102.5, -59.1784) -> (-112.5, -53.4049)
  line L731 (-112.5, -53.4049) -> (-122.5, -59.1784)
  line L732 (-122.5, -59.1784) -> (-122.5, -70.7254)
  line L733 (-122.5, -70.7254) -> (-112.5, -76.4989)
  line L734 (-87.5, -76.4989) -> (-77.5, -70.7254)
  line L735 (-77.5, -70.7254) -> (-77.5, -59.1784)
  line L736 (-77.5, -59.1784) -> (-87.5, -53.4049)
  line L737 (-87.5, -53.4049) -> (-97.5, -59.1784)
  line L738 (-97.5, -59.1784) -> (-97.5, -70.7254)
  line L739 (-97.5, -70.7254) -> (-87.5, -76.4989)
  line L740 (-62.5, -76.4989) -> (-52.5, -70.7254)
  line L741 (-52.5, -70.7254) -> (-52.5, -59.1784)
  line L742 (-52.5, -59.1784) -> (-62.5, -53.4049)
  line L743 (-62.5, -53.4049) -> (-72.5, -59.1784)
  line L744 (-72.5, -59.1784) -> (-72.5, -70.7254)
  line L745 (-72.5, -70.7254) -> (-62.5, -76.4989)
  line L746 (-37.5, -76.4989) -> (-27.5, -70.7254)
  line L747 (-27.5, -70.7254) -> (-27.5, -59.1784)
  line L748 (-27.5, -59.1784) -> (-37.5, -53.4049)
  line L749 (-37.5, -53.4049) -> (-47.5, -59.1784)
  line L750 (-47.5, -59.1784) -> (-47.5, -70.7254)
  line L751 (-47.5, -70.7254) -> (-37.5, -76.4989)
  line L752 (-12.5, -76.4989) -> (-2.5, -70.7254)
  line L753 (-2.5, -70.7254) -> (-2.5, -59.1784)
  line L754 (-2.5, -59.1784) -> (-12.5, -53.4049)
  line L755 (-12.5, -53.4049) -> (-22.5, -59.1784)
  line L756 (-22.5, -59.1784) -> (-22.5, -70.7254)
  line L757 (-22.5, -70.7254) -> (-12.5, -76.4989)
  line L758 (12.5, -76.4989) -> (22.5, -70.7254)
  line L759 (22.5, -70.7254) -> (22.5, -59.1784)
  line L760 (22.5, -59.1784) -> (12.5, -53.4049)
  line L761 (12.5, -53.4049) -> (2.5, -59.1784)
  line L762 (2.5, -59.1784) -> (2.5, -70.7254)
  line L763 (2.5, -70.7254) -> (12.5, -76.4989)
  line L764 (37.5, -76.4989) -> (47.5, -70.7254)
  line L765 (47.5, -70.7254) -> (47.5, -59.1784)
  line L766 (47.5, -59.1784) -> (37.5, -53.4049)
  line L767 (37.5, -53.4049) -> (27.5, -59.1784)
  line L768 (27.5, -59.1784) -> (27.5, -70.7254)
  line L769 (27.5, -70.7254) -> (37.5, -76.4989)
  line L770 (62.5, -76.4989) -> (72.5, -70.7254)
  line L771 (72.5, -70.7254) -> (72.5, -59.1784)
  line L772 (72.5, -59.1784) -> (62.5, -53.4049)
  line L773 (62.5, -53.4049) -> (52.5, -59.1784)
  line L774 (52.5, -59.1784) -> (52.5, -70.7254)
  line L775 (52.5, -70.7254) -> (62.5, -76.4989)
  line L776 (87.5, -76.4989) -> (97.5, -70.7254)
  line L777 (97.5, -70.7254) -> (97.5, -59.1784)
  line L778 (97.5, -59.1784) -> (87.5, -53.4049)
  line L779 (87.5, -53.4049) -> (77.5, -59.1784)
  line L780 (77.5, -59.1784) -> (77.5, -70.7254)
  line L781 (77.5, -70.7254) -> (87.5, -76.4989)
  line L782 (112.5, -76.4989) -> (122.5, -70.7254)
  line L783 (122.5, -70.7254) -> (122.5, -59.1784)
  line L784 (122.5, -59.1784) -> (112.5, -53.4049)
  line L785 (112.5, -53.4049) -> (102.5, -59.1784)
  line L786 (102.5, -59.1784) -> (102.5, -70.7254)
  line L787 (102.5, -70.7254) -> (112.5, -76.4989)
  line L788 (137.5, -76.4989) -> (147.5, -70.7254)
  line L789 (147.5, -70.7254) -> (147.5, -59.1784)
  line L790 (147.5, -59.1784) -> (137.5, -53.4049)
  line L791 (137.5, -53.4049) -> (127.5, -59.1784)
  line L792 (127.5, -59.1784) -> (127.5, -70.7254)
  line L793 (127.5, -70.7254) -> (137.5, -76.4989)
  line L794 (162.5, -76.4989) -> (172.5, -70.7254)
  line L795 (172.5, -70.7254) -> (172.5, -59.1784)
  line L796 (172.5, -59.1784) -> (162.5, -53.4049)
  line L797 (162.5, -53.4049) -> (152.5, -59.1784)
  line L798 (152.5, -59.1784) -> (152.5, -70.7254)
  line L799 (152.5, -70.7254) -> (162.5, -76.4989)
  line L800 (187.5, -76.4989) -> (197.5, -70.7254)
  line L801 (197.5, -70.7254) -> (197.5, -59.1784)
  line L802 (197.5, -59.1784) -> (187.5, -53.4049)
  line L803 (187.5, -53.4049) -> (177.5, -59.1784)
  line L804 (177.5, -59.1784) -> (177.5, -70.7254)
  line L805 (177.5, -70.7254) -> (187.5, -76.4989)
  line L806 (212.5, -76.4989) -> (222.5, -70.7254)
  line L807 (222.5, -70.7254) -> (222.5, -59.1784)
  line L808 (222.5, -59.1784) -> (212.5, -53.4049)
  line L809 (212.5, -53.4049) -> (202.5, -59.1784)
  line L810 (202.5, -59.1784) -> (202.5, -70.7254)
  line L811 (202.5, -70.7254) -> (212.5, -76.4989)
  line L812 (-125, -98.1495) -> (-115, -92.376)
  line L813 (-115, -92.376) -> (-115, -80.829)
  line L814 (-115, -80.829) -> (-125, -75.0555)
  line L815 (-125, -75.0555) -> (-135, -80.829)
  line L816 (-135, -80.829) -> (-135, -92.376)
  line L817 (-135, -92.376) -> (-125, -98.1495)
  line L818 (-100, -98.1495) -> (-90, -92.376)
  line L819 (-90, -92.376) -> (-90, -80.829)
  line L820 (-90, -80.829) -> (-100, -75.0555)
  line L821 (-100, -75.0555) -> (-110, -80.829)
  line L822 (-110, -80.829) -> (-110, -92.376)
  line L823 (-110, -92.376) -> (-100, -98.1495)
  line L824 (-75, -98.1495) -> (-65, -92.376)
  line L825 (-65, -92.376) -> (-65, -80.829)
  line L826 (-65, -80.829) -> (-75, -75.0555)
  line L827 (-75, -75.0555) -> (-85, -80.829)
  line L828 (-85, -80.829) -> (-85, -92.376)
  line L829 (-85, -92.376) -> (-75, -98.1495)
  line L830 (-50, -98.1495) -> (-40, -92.376)
  line L831 (-40, -92.376) -> (-40, -80.829)
  line L832 (-40, -80.829) -> (-50, -75.0555)
  line L833 (-50, -75.0555) -> (-60, -80.829)
  line L834 (-60, -80.829) -> (-60, -92.376)
  line L835 (-60, -92.376) -> (-50, -98.1495)
  line L836 (-25, -98.1495) -> (-15, -92.376)
  line L837 (-15, -92.376) -> (-15, -80.829)
  line L838 (-15, -80.829) -> (-25, -75.0555)
  line L839 (-25, -75.0555) -> (-35, -80.829)
  line L840 (-35, -80.829) -> (-35, -92.376)
  line L841 (-35, -92.376) -> (-25, -98.1495)
  line L842 (0, -98.1495) -> (10, -92.376)
  line L843 (10, -92.376) -> (10, -80.829)
  line L844 (10, -80.829) -> (0, -75.0555)
  line L845 (0, -75.0555) -> (-10, -80.829)
  line L846 (-10, -80.829) -> (-10, -92.376)
  line L847 (-10, -92.376) -> (0, -98.1495)
  line L848 (25, -98.1495) -> (35, -92.376)
  line L849 (35, -92.376) -> (35, -80.829)
  line L850 (35, -80.829) -> (25, -75.0555)
  line L851 (25, -75.0555) -> (15, -80.829)
  line L852 (15, -80.829) -> (15, -92.376)
  line L853 (15, -92.376) -> (25, -98.1495)
  line L854 (50, -98.1495) -> (60, -92.376)
  line L855 (60, -92.376) -> (60, -80.829)
  line L856 (60, -80.829) -> (50, -75.0555)
  line L857 (50, -75.0555) -> (40, -80.829)
  line L858 (40, -80.829) -> (40, -92.376)
  line L859 (40, -92.376) -> (50, -98.1495)
  line L860 (75, -98.1495) -> (85, -92.376)
  line L861 (85, -92.376) -> (85, -80.829)
  line L862 (85, -80.829) -> (75, -75.0555)
  line L863 (75, -75.0555) -> (65, -80.829)
  line L864 (65, -80.829) -> (65, -92.376)
  line L865 (65, -92.376) -> (75, -98.1495)
  line L866 (100, -98.1495) -> (110, -92.376)
  line L867 (110, -92.376) -> (110, -80.829)
  line L868 (110, -80.829) -> (100, -75.0555)
  line L869 (100, -75.0555) -> (90, -80.829)
  line L870 (90, -80.829) -> (90, -92.376)
  line L871 (90, -92.376) -> (100, -98.1495)
  line L872 (125, -98.1495) -> (135, -92.376)
  line L873 (135, -92.376) -> (135, -80.829)
  line L874 (135, -80.829) -> (125, -75.0555)
  line L875 (125, -75.0555) -> (115, -80.829)
  line L876 (115, -80.829) -> (115, -92.376)
  line L877 (115, -92.376) -> (125, -98.1495)
  line L878 (150, -98.1495) -> (160, -92.376)
  line L879 (160, -92.376) -> (160, -80.829)
  line L880 (160, -80.829) -> (150, -75.0555)
  line L881 (150, -75.0555) -> (140, -80.829)
  line L882 (140, -80.829) -> (140, -92.376)
  line L883 (140, -92.376) -> (150, -98.1495)
  line L884 (175, -98.1495) -> (185, -92.376)
  line L885 (185, -92.376) -> (185, -80.829)
  line L886 (185, -80.829) -> (175, -75.0555)
  line L887 (175, -75.0555) -> (165, -80.829)
  line L888 (165, -80.829) -> (165, -92.376)
  line L889 (165, -92.376) -> (175, -98.1495)
  line L890 (200, -98.1495) -> (210, -92.376)
  line L891 (210, -92.376) -> (210, -80.829)
  line L892 (210, -80.829) -> (200, -75.0555)
  line L893 (200, -75.0555) -> (190, -80.829)
  line L894 (190, -80.829) -> (190, -92.376)
  line L895 (190, -92.376) -> (200, -98.1495)
  line L896 (225, -98.1495) -> (235, -92.376)
  line L897 (235, -92.376) -> (235, -80.829)
  line L898 (235, -80.829) -> (225, -75.0555)
  line L899 (225, -75.0555) -> (215, -80.829)
  line L900 (215, -80.829) -> (215, -92.376)
  line L901 (215, -92.376) -> (225, -98.1495)
  line L902 (-112.5, -119.8002) -> (-102.5, -114.0267)
  line L903 (-102.5, -114.0267) -> (-102.5, -102.4797)
  line L904 (-102.5, -102.4797) -> (-112.5, -96.7062)
  line L905 (-112.5, -96.7062) -> (-122.5, -102.4797)
  line L906 (-122.5, -102.4797) -> (-122.5, -114.0267)
  line L907 (-122.5, -114.0267) -> (-112.5, -119.8002)
  line L908 (-87.5, -119.8002) -> (-77.5, -114.0267)
  line L909 (-77.5, -114.0267) -> (-77.5, -102.4797)
  line L910 (-77.5, -102.4797) -> (-87.5, -96.7062)
  line L911 (-87.5, -96.7062) -> (-97.5, -102.4797)
  line L912 (-97.5, -102.4797) -> (-97.5, -114.0267)
  line L913 (-97.5, -114.0267) -> (-87.5, -119.8002)
  line L914 (-62.5, -119.8002) -> (-52.5, -114.0267)
  line L915 (-52.5, -114.0267) -> (-52.5, -102.4797)
  line L916 (-52.5, -102.4797) -> (-62.5, -96.7062)
  line L917 (-62.5, -96.7062) -> (-72.5, -102.4797)
  line L918 (-72.5, -102.4797) -> (-72.5, -114.0267)
  line L919 (-72.5, -114.0267) -> (-62.5, -119.8002)
  line L920 (-37.5, -119.8002) -> (-27.5, -114.0267)
  line L921 (-27.5, -114.0267) -> (-27.5, -102.4797)
  line L922 (-27.5, -102.4797) -> (-37.5, -96.7062)
  line L923 (-37.5, -96.7062) -> (-47.5, -102.4797)
  line L924 (-47.5, -102.4797) -> (-47.5, -114.0267)
  line L925 (-47.5, -114.0267) -> (-37.5, -119.8002)
  line L926 (-12.5, -119.8002) -> (-2.5, -114.0267)
  line L927 (-2.5, -114.0267) -> (-2.5, -102.4797)
  line L928 (-2.5, -102.4797) -> (-12.5, -96.7062)
  line L929 (-12.5, -96.7062) -> (-22.5, -102.4797)
  line L930 (-22.5, -102.4797) -> (-22.5, -114.0267)
  line L931 (-22.5, -114.0267) -> (-12.5, -119.8002)
  line L932 (12.5, -119.8002) -> (22.5, -114.0267)
  line L933 (22.5, -114.0267) -> (22.5, -102.4797)
  line L934 (22.5, -102.4797) -> (12.5, -96.7062)
  line L935 (12.5, -96.7062) -> (2.5, -102.4797)
  line L936 (2.5, -102.4797) -> (2.5, -114.0267)
  line L937 (2.5, -114.0267) -> (12.5, -119.8002)
  line L938 (37.5, -119.8002) -> (47.5, -114.0267)
  line L939 (47.5, -114.0267) -> (47.5, -102.4797)
  line L940 (47.5, -102.4797) -> (37.5, -96.7062)
  line L941 (37.5, -96.7062) -> (27.5, -102.4797)
  line L942 (27.5, -102.4797) -> (27.5, -114.0267)
  line L943 (27.5, -114.0267) -> (37.5, -119.8002)
  line L944 (62.5, -119.8002) -> (72.5, -114.0267)
  line L945 (72.5, -114.0267) -> (72.5, -102.4797)
  line L946 (72.5, -102.4797) -> (62.5, -96.7062)
  line L947 (62.5, -96.7062) -> (52.5, -102.4797)
  line L948 (52.5, -102.4797) -> (52.5, -114.0267)
  line L949 (52.5, -114.0267) -> (62.5, -119.8002)
  line L950 (87.5, -119.8002) -> (97.5, -114.0267)
  line L951 (97.5, -114.0267) -> (97.5, -102.4797)
  line L952 (97.5, -102.4797) -> (87.5, -96.7062)
  line L953 (87.5, -96.7062) -> (77.5, -102.4797)
  line L954 (77.5, -102.4797) -> (77.5, -114.0267)
  line L955 (77.5, -114.0267) -> (87.5, -119.8002)
  line L956 (112.5, -119.8002) -> (122.5, -114.0267)
  line L957 (122.5, -114.0267) -> (122.5, -102.4797)
  line L958 (122.5, -102.4797) -> (112.5, -96.7062)
  line L959 (112.5, -96.7062) -> (102.5, -102.4797)
  line L960 (102.5, -102.4797) -> (102.5, -114.0267)
  line L961 (102.5, -114.0267) -> (112.5, -119.8002)
  line L962 (137.5, -119.8002) -> (147.5, -114.0267)
  line L963 (147.5, -114.0267) -> (147.5, -102.4797)
  line L964 (147.5, -102.4797) -> (137.5, -96.7062)
  line L965 (137.5, -96.7062) -> (127.5, -102.4797)
  line L966 (127.5, -102.4797) -> (127.5, -114.0267)
  line L967 (127.5, -114.0267) -> (137.5, -119.8002)
  line L968 (162.5, -119.8002) -> (172.5, -114.0267)
  line L969 (172.5, -114.0267) -> (172.5, -102.4797)
  line L970 (172.5, -102.4797) -> (162.5, -96.7062)
  line L971 (162.5, -96.7062) -> (152.5, -102.4797)
  line L972 (152.5, -102.4797) -> (152.5, -114.0267)
  line L973 (152.5, -114.0267) -> (162.5, -119.8002)
  line L974 (187.5, -119.8002) -> (197.5, -114.0267)
  line L975 (197.5, -114.0267) -> (197.5, -102.4797)
  line L976 (197.5, -102.4797) -> (187.5, -96.7062)
  line L977 (187.5, -96.7062) -> (177.5, -102.4797)
  line L978 (177.5, -102.4797) -> (177.5, -114.0267)
  line L979 (177.5, -114.0267) -> (187.5, -119.8002)
  line L980 (212.5, -119.8002) -> (222.5, -114.0267)
  line L981 (222.5, -114.0267) -> (222.5, -102.4797)
  line L982 (222.5, -102.4797) -> (212.5, -96.7062)
  line L983 (212.5, -96.7062) -> (202.5, -102.4797)
  line L984 (202.5, -102.4797) -> (202.5, -114.0267)
  line L985 (202.5, -114.0267) -> (212.5, -119.8002)
  line L986 (237.5, -119.8002) -> (247.5, -114.0267)
  line L987 (247.5, -114.0267) -> (247.5, -102.4797)
  line L988 (247.5, -102.4797) -> (237.5, -96.7062)
  line L989 (237.5, -96.7062) -> (227.5, -102.4797)